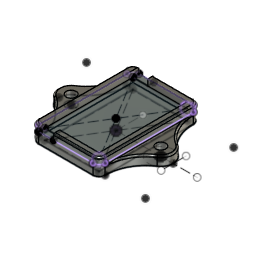
降压模块安装座-可编辑 (Autodesk Fusion 360 design; units mm, degrees)
Autodesk Fusion 360 part; units mm, degrees
sketch "草图1" plane through (0, 0, 0) normal (0, 0, 1) x (1, 0, 0)
  line L0 (8.85, 14.5) -> (-8.85, 14.5) construction
  line L1 (-8.85, 14.5) -> (-8.85, -14.5) construction
  line L2 (-8.85, -14.5) -> (8.85, -14.5) construction
  line L3 (8.85, -14.5) -> (8.85, 14.5) construction
  line L4 (8.85, 14.5) -> (-8.85, -14.5) construction
  line L5 (-8.85, 14.5) -> (8.85, -14.5) construction
  line L6 (9.1, 14.75) -> (-9.1, 14.75)
  line L7 (-9.1, 14.75) -> (-9.1, -14.75)
  line L8 (-9.1, -14.75) -> (9.1, -14.75)
  line L9 (9.1, -14.75) -> (9.1, 14.75)
  line L10 (9.1, 14.75) -> (-9.1, -14.75) construction
  line L11 (-9.1, 14.75) -> (9.1, -14.75) construction
  line L12 (-9.1, -16.75) -> (9.1, -16.75)
  line L13 (11.1, -14.75) -> (11.1, 14.75)
  line L14 (9.1, 16.75) -> (-9.1, 16.75)
  line L15 (-11.1, 14.75) -> (-11.1, -14.75)
  arc A0 (-9.1, 16.75) -> (-11.1, 14.75) centre (-9.1, 14.75) ccw
  arc A1 (11.1, 14.75) -> (9.1, 16.75) centre (9.1, 14.75) ccw
  arc A2 (9.1, -16.75) -> (11.1, -14.75) centre (9.1, -14.75) ccw
  arc A3 (-11.1, -14.75) -> (-9.1, -16.75) centre (-9.1, -14.75) ccw
  circle A4 centre (15, 0) radius 1.65
  line L16 (0, 0) -> (0, 9) construction
  circle A5 centre (-15, 0) radius 1.65
  line L17 (19.1, 4.3337) -> (19.1, -4) construction
  circle A6 centre (15, 0) radius 4.1 construction
  arc A7 (11.1, 14.75) -> (17.2361, 3.4365) centre (24.5977, 14.75) ccw
  arc A8 (19.1, 0) -> (17.2361, 3.4365) centre (15, 0) ccw
  line L18 (0, 0) -> (27.1496, 0) construction
  arc A9 (17.2361, -3.4365) -> (11.1, -14.75) centre (24.5977, -14.75) ccw
  arc A10 (17.2361, -3.4365) -> (19.1, 0) centre (15, 0) ccw
  arc A11 (-17.2361, 3.4365) -> (-11.1, 14.75) centre (-24.5977, 14.75) ccw
  arc A12 (-17.2361, 3.4365) -> (-19.1, 0) centre (-15, 0) ccw
  arc A13 (-19.1, 0) -> (-17.2361, -3.4365) centre (-15, 0) ccw
  arc A14 (-11.1, -14.75) -> (-17.2361, -3.4365) centre (-24.5977, -14.75) ccw
  dimension "d1" = 17.7
  dimension "d2" = 29
  dimension "d3" = 18.2
  dimension "d4" = 29.5
  dimension "d8" = 2
  dimension "d17" = 3.3
  dimension "d18" = 15
  dimension "d19" = 8
  constraint horizontal L0
  constraint perpendicular L0 L1
  constraint parallel L0 L2
  constraint parallel L1 L3
  constraint coincident L4 L16.start
  constraint coincident L5 L16.start
  constraint coincident L16.start L18.start
  constraint horizontal L6
  constraint perpendicular L6 L7
  constraint parallel L6 L8
  constraint parallel L7 L9
  constraint coincident L10 L16.start
  constraint coincident L11 L16.start
  constraint tangent L14 A0
  constraint tangent L15 A0
  constraint tangent L13 A1
  constraint tangent L14 A1
  constraint equal A0 A1
  constraint tangent L12 A2
  constraint tangent L13 A2
  constraint equal A0 A2
  constraint tangent L12 A3
  constraint tangent L15 A3
  constraint equal A0 A3
  constraint vertical L16
  constraint symmetric A4 L16 A5
  constraint horizontal L16.start A4.centre
  constraint parallel L13 L17
  constraint tangent L17 A6
  constraint tangent A6 A7
  constraint tangent L13 A7
  constraint horizontal L6.start A7.centre
  constraint coincident A6 A7.end
  constraint coincident A4.centre A6.centre
  constraint coincident A6 A8.start
  constraint tangent A7 A8
  constraint horizontal L18
  constraint symmetric L13.end L18 L13.start
  constraint symmetric A7 L18 A9
  constraint symmetric A7.end L18 A9.start
  constraint symmetric A8.start L18 A10.end
  constraint symmetric A8 L18 A10
  constraint symmetric L13.end L16 L15.start
  constraint symmetric L16 A7 A11
  constraint symmetric L16 A7.end A11.start
  constraint symmetric L16 A8.start A12.end
  constraint symmetric L16 A8 A12
  constraint symmetric L16 L13.start L15.end
  constraint symmetric L16 A9.start A13.end
  constraint symmetric L16 A9 A14
  constraint symmetric L16 A10 A13
  measures "d1" distance of L1.end L2.end
  measures "d2" distance of L0.end L1.end
  measures "d3" distance of L7.end L8.end
  measures "d4" distance of L6.end L7.end
  measures "d8" radius of A0
  measures "d17" diameter of A4
  measures "d18" distance of L16.start A4.centre
  measures "d19" distance of L13 L17
extrude "拉伸1" add sketch "草图1" along normal blind 3.5 contours L6 L7 L8 L9 | L12 L13 L14 L15 A0 A1 A2 A3 makes body 1
sketch "草图2" plane through (0, 0, 3.5) normal (0, 0, 1) x (-1, 0, 0)
  line L0 (11.1, -14.75) -> (11.1, 14.75)
  line L1 (9.1, 16.75) -> (-9.1, 16.75)
  line L2 (-11.1, 14.75) -> (-11.1, -14.75)
  line L3 (-9.1, -16.75) -> (9.1, -16.75)
  arc A0 (11.1, 14.75) -> (9.1, 16.75) centre (9.1, 14.75) ccw
  arc A1 (-9.1, 16.75) -> (-11.1, 14.75) centre (-9.1, 14.75) ccw
  arc A2 (-11.1, -14.75) -> (-9.1, -16.75) centre (-9.1, -14.75) ccw
  arc A3 (9.1, -16.75) -> (11.1, -14.75) centre (9.1, -14.75) ccw
  line L4 (-9.1, -14.75) -> (9.1, -14.75)
  line L5 (9.1, -14.75) -> (9.1, 14.75)
  line L6 (9.1, 14.75) -> (-9.1, 14.75)
  line L7 (-9.1, 14.75) -> (-9.1, -14.75)
  line L8 (-9.1, -14.75) -> (9.1, 14.75) construction
  line L9 (9.1, -14.75) -> (-9.1, 14.75) construction
  line L10 (9.1, -14.75) -> (9.1, -16.75)
  line L11 (4.1, -14.75) -> (4.1, -16.75)
  line L12 (9.1, 14.75) -> (9.1, 16.75)
  line L13 (4.1, 14.75) -> (4.1, 16.75)
  dimension "d9" = 18.2
  dimension "d10" = 29.5
  dimension "d11" = 5
  dimension "d12" = 5
  constraint horizontal L4
  constraint perpendicular L4 L5
  constraint parallel L4 L6
  constraint parallel L5 L7
  constraint coincident L8 origin
  constraint coincident L9 origin
  constraint coincident A3.centre L4.end
  constraint coincident L3.end A3.start
  constraint coincident L4 L11.start
  constraint coincident L3 L11.end
  constraint perpendicular L3 L11
  constraint coincident A0.centre L5.end
  constraint coincident L1.start A0.end
  constraint coincident L6 L13.start
  constraint coincident L1 L13.end
  constraint perpendicular L1 L13
  measures "d9" distance of A0.centre A1.centre
  measures "d10" distance of A3.centre A0.centre
  measures "d11" distance of L10 L11
  measures "d12" distance of L12 L13
extrude "拉伸2" add sketch "草图2" along normal blind 2 contours L0 A0 A3 L5 L10 L12 | L1 L2 L3 A1 A2 L4 L6 L7 L11 L13 bodies 1
extrude "拉伸3" cut sketch "草图2" against normal blind 1.5 contours L4 L5 L6 L7 bodies 1
extrude "拉伸4" add sketch "草图1" along normal blind 3 separate body contours L15 A11 A12 A13 A14 | L13 A7 A8 A9 A10 makes body 2 at (-11.1, 4.9167, 1) makes body 3 at (11.1, -4.9167, 1)
fillet "圆角1" radius 0.5 3 edges at (-12.7328, 8.3148, 3) (-19.1, 0, 3) (-12.7328, -8.3148, 3) on bodies 2
fillet "圆角2" radius 0.5 11 edges at (2.5, -16.75, 5.5) (10.5142, -16.1642, 5.5) (11.1, 0, 5.5) (10.5142, 16.1642, 5.5) (2.5, 16.75, 5.5) (-10.5142, 16.1642, 5.5) (-11.1, 0, 5.5) (-10.5142, -16.1642, 5.5) (12.7328, -8.3148, 3) (19.1, 0, 3) (12.7328, 8.3148, 3) on bodies 1 3
equation "d3 = 17.7 mm + 0.5 mm"
equation "d6 = 1.5 mm + 2 mm"
